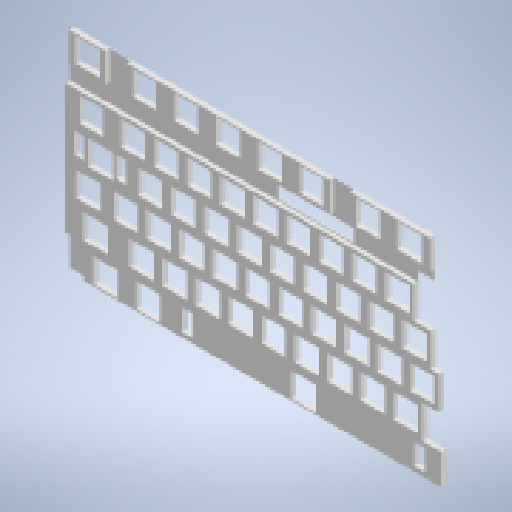
# Autodesk Inventor part: Left plate
Saved by Autodesk Inventor 2025 (Build 290162000, 162)
## iProperties
Created: 2024-08-01
Part Number: Left plate
Material: PET Plastic
Document SubType Name: Modeling
Designer: adam
Density: 1.541 g/cm^3
Appearance: White
Author: adam
Autodesk Inventor part; units mm, degrees
(part 1 of 2)
ref_plane "YZ Plane" through (0, 0, 0) normal (1, 0, 0) x (0, 1, 0)
ref_plane "XZ Plane" through (0, 0, 0) normal (0, 1, 0) x (-1, 0, 0)
ref_plane "XY Plane" through (0, 0, 0) normal (0, 0, 1) x (1, 0, 0)
sketch "Sketch3" plane through (0, 0, 0) normal (0, 0, 1) x (1, 0, 0)
  line L0 (316, -123) -> (0, -123) construction
  line L1 (316, -2) -> (316, -123) construction
  line L2 (0, -2) -> (316, -2) construction
  line L3 (0, -123) -> (0, -2) construction
  circle A0 centre (18.6, -119.6) radius 0.725 construction
  circle A1 centre (23, -114.9) radius 2.55 construction
  circle A2 centre (25.6, -120.65) radius 0.725 construction
  circle A3 centre (43.1, -119.6) radius 0.725 construction
  circle A4 centre (50.1, -120.65) radius 0.725 construction
  circle A5 centre (47.5, -114.9) radius 2.55 construction
  line L4 (67.3517, -120.975) -> (73.3517, -120.975) construction
  line L5 (67.3517, -105.975) -> (67.3517, -120.975) construction
  line L6 (73.3517, -105.975) -> (67.3517, -105.975) construction
  line L7 (73.3517, -120.975) -> (73.3517, -105.975) construction
  circle A6 centre (13.1, -100.5) radius 0.725 construction
  circle A7 centre (20.1, -101.55) radius 0.725 construction
  circle A8 centre (39.35, -100.5) radius 0.725 construction
  circle A9 centre (17.5, -95.8) radius 2.55 construction
  circle A10 centre (46.35, -101.55) radius 0.725 construction
  circle A11 centre (58.35, -100.5) radius 0.725 construction
  circle A12 centre (65.35, -101.55) radius 0.725 construction
  circle A13 centre (77.35, -100.5) radius 0.725 construction
  circle A14 centre (43.75, -95.8) radius 2.55 construction
  circle A15 centre (62.75, -95.8) radius 2.55 construction
  circle A16 centre (81.75, -95.8) radius 2.55 construction
  circle A17 centre (132.4518, -119.675) radius 0.725 construction
  circle A18 centre (139.4518, -120.725) radius 0.725 construction
  circle A19 centre (136.8518, -114.975) radius 2.55 construction
  circle A20 centre (84.35, -101.55) radius 0.725 construction
  circle A21 centre (96.35, -100.5) radius 0.725 construction
  circle A22 centre (103.35, -101.55) radius 0.725 construction
  circle A23 centre (115.35, -100.5) radius 0.725 construction
  circle A24 centre (100.75, -95.8) radius 2.55 construction
  circle A25 centre (119.75, -95.8) radius 2.55 construction
  circle A26 centre (122.35, -101.55) radius 0.725 construction
  circle A27 centre (134.35, -100.5) radius 0.725 construction
  circle A28 centre (141.35, -101.55) radius 0.725 construction
  circle A29 centre (153.35, -100.5) radius 0.725 construction
  circle A30 centre (138.75, -95.8) radius 2.55 construction
  circle A31 centre (157.75, -95.8) radius 2.55 construction
  circle A32 centre (15.6, -82.45) radius 0.725 construction
  circle A33 centre (8.6, -81.4) radius 0.725 construction
  circle A34 centre (37.1, -82.45) radius 0.725 construction
  circle A35 centre (30.1, -81.4) radius 0.725 construction
  circle A36 centre (56.1, -82.45) radius 0.725 construction
  circle A37 centre (49.1, -81.4) radius 0.725 construction
  circle A38 centre (75.1, -82.45) radius 0.725 construction
  circle A39 centre (68.1, -81.4) radius 0.725 construction
  circle A40 centre (13, -76.7) radius 2.55 construction
  circle A41 centre (34.5, -76.7) radius 2.55 construction
  circle A42 centre (53.5, -76.7) radius 2.55 construction
  circle A43 centre (72.5, -76.7) radius 2.55 construction
  circle A44 centre (94.1, -82.45) radius 0.725 construction
  circle A45 centre (87.1, -81.4) radius 0.725 construction
  circle A46 centre (113.1, -82.45) radius 0.725 construction
  circle A47 centre (106.1, -81.4) radius 0.725 construction
  circle A48 centre (132.1, -82.45) radius 0.725 construction
  circle A49 centre (125.1, -81.4) radius 0.725 construction
  circle A50 centre (151.1, -82.45) radius 0.725 construction
  circle A51 centre (144.1, -81.4) radius 0.725 construction
  circle A52 centre (91.5, -76.7) radius 2.55 construction
  circle A53 centre (110.5, -76.7) radius 2.55 construction
  circle A54 centre (129.5, -76.7) radius 2.55 construction
  circle A55 centre (148.5, -76.7) radius 2.55 construction
  circle A56 centre (221.85, -119.6) radius 0.725 construction
  circle A57 centre (228.85, -120.65) radius 0.725 construction
  circle A58 centre (226.25, -114.9) radius 2.55 construction
  line L8 (200.3518, -120.975) -> (206.3518, -120.975) construction
  line L9 (200.3518, -105.975) -> (200.3518, -120.975) construction
  line L10 (206.3518, -105.975) -> (200.3518, -105.975) construction
  line L11 (206.3518, -120.975) -> (206.3518, -105.975) construction
  circle A59 centre (160.35, -101.55) radius 0.725 construction
  circle A60 centre (172.35, -100.5) radius 0.725 construction
  circle A61 centre (179.35, -101.55) radius 0.725 construction
  circle A62 centre (191.35, -100.5) radius 0.725 construction
  circle A63 centre (198.35, -101.55) radius 0.725 construction
  circle A64 centre (176.75, -95.8) radius 2.55 construction
  circle A65 centre (195.75, -95.8) radius 2.55 construction
  circle A66 centre (210.35, -100.5) radius 0.725 construction
  circle A67 centre (217.35, -101.55) radius 0.725 construction
  circle A68 centre (229.35, -100.5) radius 0.725 construction
  circle A69 centre (236.35, -101.55) radius 0.725 construction
  circle A70 centre (214.75, -95.8) radius 2.55 construction
  circle A71 centre (233.75, -95.8) radius 2.55 construction
  circle A72 centre (243.85, -119.6) radius 0.725 construction
  circle A73 centre (250.85, -120.65) radius 0.725 construction
  circle A74 centre (248.25, -114.9) radius 2.55 construction
  circle A75 centre (262.85, -119.6) radius 0.725 construction
  circle A76 centre (269.85, -120.65) radius 0.725 construction
  circle A77 centre (267.25, -114.9) radius 2.55 construction
  circle A78 centre (281.85, -119.6) radius 0.725 construction
  circle A79 centre (288.85, -120.65) radius 0.725 construction
  circle A80 centre (286.25, -114.9) radius 2.55 construction
  circle A81 centre (300.85, -119.6) radius 0.725 construction
  circle A82 centre (307.85, -120.65) radius 0.725 construction
  circle A83 centre (305.25, -114.9) radius 2.55 construction
  circle A84 centre (255.6, -100.5) radius 0.725 construction
  circle A85 centre (262.6, -101.55) radius 0.725 construction
  circle A86 centre (260, -95.8) radius 2.55 construction
  circle A87 centre (281.85, -100.5) radius 0.725 construction
  circle A88 centre (288.85, -101.55) radius 0.725 construction
  circle A89 centre (314, -102.5) radius 0.5 construction
  circle A90 centre (286.25, -95.8) radius 2.55 construction
  circle A91 centre (314, -99.96) radius 0.5 construction
  circle A92 centre (314, -97.42) radius 0.5 construction
  circle A93 centre (314, -94.88) radius 0.5 construction
  circle A94 centre (170.1, -82.45) radius 0.725 construction
  circle A95 centre (163.1, -81.4) radius 0.725 construction
  circle A96 centre (189.1, -82.45) radius 0.725 construction
  circle A97 centre (182.1, -81.4) radius 0.725 construction
  circle A98 centre (208.1, -82.45) radius 0.725 construction
  circle A99 centre (201.1, -81.4) radius 0.725 construction
  circle A100 centre (227.1, -82.45) radius 0.725 construction
  circle A101 centre (220.1, -81.4) radius 0.725 construction
  circle A102 centre (167.5, -76.7) radius 2.55 construction
  circle A103 centre (186.5, -76.7) radius 2.55 construction
  circle A104 centre (205.5, -76.7) radius 2.55 construction
  circle A105 centre (224.5, -76.7) radius 2.55 construction
  circle A106 centre (246.1, -82.45) radius 0.725 construction
  circle A107 centre (239.1, -81.4) radius 0.725 construction
  circle A108 centre (265.1, -82.45) radius 0.725 construction
  circle A109 centre (258.1, -81.4) radius 0.725 construction
  circle A110 centre (314, -92.34) radius 0.5 construction
  circle A111 centre (314, -89.8) radius 0.5 construction
  line L12 (275, -82.25) -> (290, -82.25) construction
  line L13 (275, -76.25) -> (275, -82.25) construction
  line L14 (290, -76.25) -> (275, -76.25) construction
  line L15 (290, -82.25) -> (290, -76.25) construction
  circle A112 centre (243.5, -76.7) radius 2.55 construction
  circle A113 centre (262.5, -76.7) radius 2.55 construction
  circle A114 centre (288.675, -71.675) radius 0.725 construction
  circle A115 centre (283.975, -67.275) radius 2.55 construction
  circle A116 centre (289.725, -64.675) radius 0.725 construction
  circle A117 centre (22.6, -63.35) radius 0.725 construction
  circle A118 centre (15.6, -62.3) radius 0.725 construction
  circle A119 centre (20, -57.6) radius 2.55 construction
  line L16 (5, -63.6) -> (11, -63.6) construction
  line L17 (5, -48.6) -> (5, -63.6) construction
  line L18 (11, -48.6) -> (5, -48.6) construction
  line L19 (11, -63.6) -> (11, -48.6) construction
  line L20 (29, -63.6) -> (35, -63.6) construction
  line L21 (29, -48.6) -> (29, -63.6) construction
  line L22 (35, -48.6) -> (29, -48.6) construction
  line L23 (35, -63.6) -> (35, -48.6) construction
  circle A120 centre (51.35, -63.35) radius 0.725 construction
  circle A121 centre (44.35, -62.3) radius 0.725 construction
  circle A122 centre (48.75, -57.6) radius 2.55 construction
  circle A123 centre (70.35, -63.35) radius 0.725 construction
  circle A124 centre (63.35, -62.3) radius 0.725 construction
  circle A125 centre (82.35, -62.3) radius 0.725 construction
  circle A126 centre (67.75, -57.6) radius 2.55 construction
  circle A127 centre (10.6, -43.2) radius 0.725 construction
  circle A128 centre (17.6, -44.25) radius 0.725 construction
  circle A129 centre (34.6, -43.2) radius 0.725 construction
  circle A130 centre (41.6, -44.25) radius 0.725 construction
  circle A131 centre (15, -38.5) radius 2.55 construction
  circle A132 centre (39, -38.5) radius 2.55 construction
  circle A133 centre (53.6, -43.2) radius 0.725 construction
  circle A134 centre (60.6, -44.25) radius 0.725 construction
  circle A135 centre (72.6, -43.2) radius 0.725 construction
  circle A136 centre (79.6, -44.25) radius 0.725 construction
  circle A137 centre (58, -38.5) radius 2.55 construction
  circle A138 centre (77, -38.5) radius 2.55 construction
  circle A139 centre (89.35, -63.35) radius 0.725 construction
  circle A140 centre (101.35, -62.3) radius 0.725 construction
  circle A141 centre (86.75, -57.6) radius 2.55 construction
  circle A142 centre (108.35, -63.35) radius 0.725 construction
  circle A143 centre (120.35, -62.3) radius 0.725 construction
  circle A144 centre (105.75, -57.6) radius 2.55 construction
  circle A145 centre (127.35, -63.35) radius 0.725 construction
  circle A146 centre (139.35, -62.3) radius 0.725 construction
  circle A147 centre (124.75, -57.6) radius 2.55 construction
  circle A148 centre (146.35, -63.35) radius 0.725 construction
  circle A149 centre (158.35, -62.3) radius 0.725 construction
  circle A150 centre (143.75, -57.6) radius 2.55 construction
  circle A151 centre (91.6, -43.2) radius 0.725 construction
  circle A152 centre (98.6, -44.25) radius 0.725 construction
  circle A153 centre (110.6, -43.2) radius 0.725 construction
  circle A154 centre (117.6, -44.25) radius 0.725 construction
  circle A155 centre (96, -38.5) radius 2.55 construction
  circle A156 centre (115, -38.5) radius 2.55 construction
  circle A157 centre (129.6, -43.2) radius 0.725 construction
  circle A158 centre (136.6, -44.25) radius 0.725 construction
  circle A159 centre (148.6, -43.2) radius 0.725 construction
  circle A160 centre (155.6, -44.25) radius 0.725 construction
  circle A161 centre (134, -38.5) radius 2.55 construction
  circle A162 centre (153, -38.5) radius 2.55 construction
  circle A163 centre (8.1, -14.7) radius 0.725 construction
  circle A164 centre (15.1, -15.75) radius 0.725 construction
  circle A165 centre (41.1, -14.7) radius 0.725 construction
  circle A166 centre (12.5, -10) radius 2.55 construction
  circle A167 centre (48.1, -15.75) radius 0.725 construction
  circle A168 centre (65.1, -14.7) radius 0.725 construction
  circle A169 centre (72.1, -15.75) radius 0.725 construction
  circle A170 centre (45.5, -10) radius 2.55 construction
  circle A171 centre (69.5, -10) radius 2.55 construction
  circle A172 centre (123.5, -26.25) radius 0.425 construction
  circle A173 centre (126, -26.25) radius 0.425 construction
  circle A174 centre (128.5, -26.25) radius 0.425 construction
  circle A175 centre (131, -26.25) radius 0.425 construction
  circle A176 centre (133.5, -26.25) radius 0.425 construction
  circle A177 centre (136, -26.25) radius 0.425 construction
  circle A178 centre (138.5, -26.25) radius 0.425 construction
  circle A179 centre (122.25, -23.75) radius 0.425 construction
  circle A180 centre (124.75, -23.75) radius 0.425 construction
  circle A181 centre (127.25, -23.75) radius 0.425 construction
  circle A182 centre (129.75, -23.75) radius 0.425 construction
  circle A183 centre (132.25, -23.75) radius 0.425 construction
  circle A184 centre (134.75, -23.75) radius 0.425 construction
  circle A185 centre (137.25, -23.75) radius 0.425 construction
  circle A186 centre (139.75, -23.75) radius 0.425 construction
  circle A187 centre (141, -26.25) radius 0.425 construction
  circle A188 centre (143.5, -26.25) radius 0.425 construction
  circle A189 centre (146, -26.25) radius 0.425 construction
  circle A190 centre (148.5, -26.25) radius 0.425 construction
  circle A191 centre (151, -26.25) radius 0.425 construction
  circle A192 centre (153.5, -26.25) radius 0.425 construction
  circle A193 centre (156, -26.25) radius 0.425 construction
  circle A194 centre (158.5, -26.25) radius 0.425 construction
  circle A195 centre (142.25, -23.75) radius 0.425 construction
  circle A196 centre (144.75, -23.75) radius 0.425 construction
  circle A197 centre (147.25, -23.75) radius 0.425 construction
  circle A198 centre (149.75, -23.75) radius 0.425 construction
  circle A199 centre (152.25, -23.75) radius 0.425 construction
  circle A200 centre (154.75, -23.75) radius 0.425 construction
  circle A201 centre (157.25, -23.75) radius 0.425 construction
  circle A202 centre (89.1, -14.7) radius 0.725 construction
  circle A203 centre (96.1, -15.75) radius 0.725 construction
  circle A204 centre (113.1, -14.7) radius 0.725 construction
  circle A205 centre (120.1, -15.75) radius 0.725 construction
  circle A206 centre (93.5, -10) radius 2.55 construction
  circle A207 centre (117.5, -10) radius 2.55 construction
  circle A208 centre (137.1, -14.7) radius 0.725 construction
  circle A209 centre (144.1, -15.75) radius 0.725 construction
  circle A210 centre (141.5, -10) radius 2.55 construction
  circle A211 centre (165.35, -63.35) radius 0.725 construction
  circle A212 centre (177.35, -62.3) radius 0.725 construction
  circle A213 centre (162.75, -57.6) radius 2.55 construction
  circle A214 centre (184.35, -63.35) radius 0.725 construction
  circle A215 centre (196.35, -62.3) radius 0.725 construction
  circle A216 centre (181.75, -57.6) radius 2.55 construction
  circle A217 centre (203.35, -63.35) radius 0.725 construction
  circle A218 centre (215.35, -62.3) radius 0.725 construction
  circle A219 centre (200.75, -57.6) radius 2.55 construction
  circle A220 centre (222.35, -63.35) radius 0.725 construction
  circle A221 centre (234.35, -62.45) radius 0.725 construction
  circle A222 centre (219.75, -57.6) radius 2.55 construction
  circle A223 centre (167.6, -43.2) radius 0.725 construction
  circle A224 centre (174.6, -44.25) radius 0.725 construction
  circle A225 centre (186.6, -43.2) radius 0.725 construction
  circle A226 centre (193.6, -44.25) radius 0.725 construction
  circle A227 centre (172, -38.5) radius 2.55 construction
  circle A228 centre (191, -38.5) radius 2.55 construction
  circle A229 centre (205.6, -43.2) radius 0.725 construction
  circle A230 centre (212.6, -44.25) radius 0.725 construction
  circle A231 centre (224.6, -43.2) radius 0.725 construction
  circle A232 centre (231.6, -44.25) radius 0.725 construction
  circle A233 centre (210, -38.5) radius 2.55 construction
  circle A234 centre (229, -38.5) radius 2.55 construction
  circle A235 centre (241.35, -63.5) radius 0.725 construction
  circle A236 centre (253.35, -62.4466) radius 0.725 construction
  circle A237 centre (238.75, -57.75) radius 2.55 construction
  circle A238 centre (260.35, -63.4966) radius 0.725 construction
  circle A239 centre (257.75, -57.7466) radius 2.55 construction
  line L24 (275, -58.25) -> (290, -58.25) construction
  line L25 (275, -52.25) -> (275, -58.25) construction
  line L26 (290, -52.25) -> (275, -52.25) construction
  line L27 (290, -58.25) -> (290, -52.25) construction
  circle A240 centre (243.6, -43.2) radius 0.725 construction
  circle A241 centre (250.6, -44.25) radius 0.725 construction
  circle A242 centre (262.6, -43.2) radius 0.725 construction
  circle A243 centre (269.6, -44.25) radius 0.725 construction
  circle A244 centre (248, -38.5) radius 2.55 construction
  circle A245 centre (267, -38.5) radius 2.55 construction
  circle A246 centre (281.6, -43.2) radius 0.725 construction
  circle A247 centre (288.6, -44.25) radius 0.725 construction
  circle A248 centre (300.6, -43.2) radius 0.725 construction
  circle A249 centre (307.6, -44.25) radius 0.725 construction
  circle A250 centre (286, -38.5) radius 2.55 construction
  circle A251 centre (305, -38.5) radius 2.55 construction
  circle A252 centre (161, -26.25) radius 0.425 construction
  circle A253 centre (159.75, -23.75) radius 0.425 construction
  circle A254 centre (219, -34) radius 1.6 construction
  circle A255 centre (169.6, -14.7) radius 0.725 construction
  circle A256 centre (176.6, -15.75) radius 0.725 construction
  circle A257 centre (193.6, -14.7) radius 0.725 construction
  circle A258 centre (174, -10) radius 2.55 construction
  circle A259 centre (198, -10) radius 2.55 construction
  circle A260 centre (200.6, -15.75) radius 0.725 construction
  circle A261 centre (217.6, -14.7) radius 0.725 construction
  circle A262 centre (224.6, -15.75) radius 0.725 construction
  circle A263 centre (222, -10) radius 2.55 construction
  circle A264 centre (241.6, -14.7) radius 0.725 construction
  circle A265 centre (248.6, -15.75) radius 0.725 construction
  circle A266 centre (265.6, -14.7) radius 0.725 construction
  circle A267 centre (272.6, -15.75) radius 0.725 construction
  circle A268 centre (246, -10) radius 2.55 construction
  circle A269 centre (270, -10) radius 2.55 construction
  circle A270 centre (299.1, -14.7) radius 0.725 construction
  circle A271 centre (306.1, -15.75) radius 0.725 construction
  circle A272 centre (303.5, -10) radius 2.55 construction
  line L28 (216.3009, -122.9025) -> (216.3009, -103.8025)
  line L29 (216.3009, -103.8025) -> (205.25, -103.8025)
  line L30 (205.25, -103.8025) -> (205.25, -86.25)
  line L31 (205.25, -86.25) -> (215, -86.25)
  line L32 (215, -86.25) -> (215, -67.15)
  line L33 (215, -67.15) -> (210.25, -67.15)
  line L34 (210.25, -67.15) -> (210.25, -48.05)
  line L35 (210.25, -48.05) -> (200.5, -48.05)
  line L36 (200.5, -48.05) -> (200.5, -24.25)
  line L37 (200.5, -24.25) -> (210, -24.25)
  line L38 (210, -24.25) -> (210, -1.9975)
  line L39 (198, -10) -> (210, -10) construction
  line L40 (210, -10) -> (222, -10) construction
  line L41 (191, -38.5) -> (200.5, -38.5) construction
  line L42 (210, -38.5) -> (200.5, -38.5) construction
  line L43 (200.75, -57.6) -> (210.25, -57.6) construction
  line L44 (219.75, -57.6) -> (210.25, -57.6) construction
  line L45 (205.5, -76.7) -> (215, -76.7) construction
  line L46 (224.5, -76.7) -> (215, -76.7) construction
  line L47 (195.75, -95.8) -> (205.25, -95.8) construction
  line L48 (214.75, -95.8) -> (205.25, -95.8) construction
  line L49 (226.25, -114.9) -> (216.3009, -114.9) construction
  line L50 (206.3518, -114.9) -> (216.3009, -114.9) construction
  line L51 (204, -10) -> (204, -24.25) construction
  line L52 (204, -38.5) -> (204, -24.25) construction
  line L53 (206.8595, -38.5) -> (206.8595, -48.05) construction
  line L54 (206.8595, -57.6) -> (206.8595, -48.05) construction
  line L55 (211.5322, -57.6) -> (211.5322, -67.15) construction
  line L56 (211.5322, -67.15) -> (211.5322, -76.7) construction
  line L57 (209.7471, -76.7) -> (209.7471, -86.25) construction
  line L58 (209.7471, -86.25) -> (209.7471, -95.8) construction
  line L59 (207.7475, -88.7975) -> (221.7525, -88.7975) construction
  line L60 (221.7525, -88.7975) -> (221.7525, -102.8025) construction
  line L61 (221.7525, -102.8025) -> (207.7475, -102.8025) construction
  line L62 (207.7475, -102.8025) -> (207.7475, -88.7975) construction
  line L63 (207.7475, -88.7975) -> (221.7525, -102.8025) construction
  line L64 (221.7525, -88.7975) -> (207.7475, -102.8025) construction
  line L65 (129.8493, -107.9725) -> (143.8543, -107.9725)
  line L66 (143.8543, -107.9725) -> (143.8543, -121.9775)
  line L67 (143.8543, -121.9775) -> (129.8493, -121.9775)
  line L68 (129.8493, -121.9775) -> (129.8493, -107.9725)
  line L69 (129.8493, -107.9725) -> (143.8543, -121.9775) construction
  line L70 (143.8543, -107.9725) -> (129.8493, -121.9775) construction
  line L71 (143.8543, -107.9725) -> (216.3009, -107.9725) construction
  line L72 (5.4975, -2.9975) -> (19.5025, -2.9975)
  line L73 (19.5025, -2.9975) -> (19.5025, -17.0025)
  line L74 (19.5025, -17.0025) -> (5.4975, -17.0025)
  line L75 (5.4975, -17.0025) -> (5.4975, -2.9975)
  line L76 (5.4975, -2.9975) -> (19.5025, -17.0025) construction
  line L77 (19.5025, -2.9975) -> (5.4975, -17.0025) construction
  line L78 (38.4975, -2.9975) -> (52.5025, -2.9975)
  line L79 (52.5025, -2.9975) -> (52.5025, -17.0025)
  line L80 (52.5025, -17.0025) -> (38.4975, -17.0025)
  line L81 (38.4975, -17.0025) -> (38.4975, -2.9975)
  line L82 (38.4975, -2.9975) -> (52.5025, -17.0025) construction
  line L83 (52.5025, -2.9975) -> (38.4975, -17.0025) construction
  line L84 (62.4975, -2.9975) -> (76.5025, -2.9975)
  line L85 (76.5025, -2.9975) -> (76.5025, -17.0025)
  line L86 (76.5025, -17.0025) -> (62.4975, -17.0025)
  line L87 (62.4975, -17.0025) -> (62.4975, -2.9975)
  line L88 (62.4975, -2.9975) -> (76.5025, -17.0025) construction
  line L89 (76.5025, -2.9975) -> (62.4975, -17.0025) construction
  line L90 (86.4975, -2.9975) -> (100.5025, -2.9975)
  line L91 (100.5025, -2.9975) -> (100.5025, -17.0025)
  line L92 (100.5025, -17.0025) -> (86.4975, -17.0025)
  line L93 (86.4975, -17.0025) -> (86.4975, -2.9975)
  line L94 (86.4975, -2.9975) -> (100.5025, -17.0025) construction
  line L95 (100.5025, -2.9975) -> (86.4975, -17.0025) construction
  line L96 (110.4975, -2.9975) -> (124.5025, -2.9975)
  line L97 (124.5025, -2.9975) -> (124.5025, -17.0025)
  line L98 (124.5025, -17.0025) -> (110.4975, -17.0025)
  line L99 (110.4975, -17.0025) -> (110.4975, -2.9975)
  line L100 (110.4975, -2.9975) -> (124.5025, -17.0025) construction
  line L101 (124.5025, -2.9975) -> (110.4975, -17.0025) construction
  line L102 (134.4975, -2.9975) -> (148.5025, -2.9975)
  line L103 (148.5025, -2.9975) -> (148.5025, -17.0025)
  line L104 (148.5025, -17.0025) -> (134.4975, -17.0025)
  line L105 (134.4975, -17.0025) -> (134.4975, -2.9975)
  line L106 (134.4975, -2.9975) -> (148.5025, -17.0025) construction
  line L107 (148.5025, -2.9975) -> (134.4975, -17.0025) construction
  line L108 (166.9975, -2.9975) -> (181.0025, -2.9975)
  line L109 (181.0025, -2.9975) -> (181.0025, -17.0025)
  line L110 (181.0025, -17.0025) -> (166.9975, -17.0025)
  line L111 (166.9975, -17.0025) -> (166.9975, -2.9975)
  line L112 (166.9975, -2.9975) -> (181.0025, -17.0025) construction
  line L113 (181.0025, -2.9975) -> (166.9975, -17.0025) construction
  line L114 (190.9975, -2.9975) -> (205.0025, -2.9975)
  line L115 (205.0025, -2.9975) -> (205.0025, -17.0025)
  line L116 (205.0025, -17.0025) -> (190.9975, -17.0025)
  line L117 (190.9975, -17.0025) -> (190.9975, -2.9975)
  line L118 (190.9975, -2.9975) -> (205.0025, -17.0025) construction
  line L119 (205.0025, -2.9975) -> (190.9975, -17.0025) construction
  line L120 (7.9975, -31.4975) -> (22.0025, -31.4975)
  line L121 (22.0025, -31.4975) -> (22.0025, -45.5025)
  line L122 (22.0025, -45.5025) -> (7.9975, -45.5025)
  line L123 (7.9975, -45.5025) -> (7.9975, -31.4975)
  line L124 (7.9975, -31.4975) -> (22.0025, -45.5025) construction
  line L125 (22.0025, -31.4975) -> (7.9975, -45.5025) construction
  line L126 (31.9975, -31.4975) -> (46.0025, -31.4975)
  line L127 (46.0025, -31.4975) -> (46.0025, -45.5025)
  line L128 (46.0025, -45.5025) -> (31.9975, -45.5025)
  line L129 (31.9975, -45.5025) -> (31.9975, -31.4975)
  line L130 (31.9975, -31.4975) -> (46.0025, -45.5025) construction
  line L131 (46.0025, -31.4975) -> (31.9975, -45.5025) construction
  line L132 (50.9975, -31.4975) -> (65.0025, -31.4975)
  line L133 (65.0025, -31.4975) -> (65.0025, -45.5025)
  line L134 (65.0025, -45.5025) -> (50.9975, -45.5025)
  line L135 (50.9975, -45.5025) -> (50.9975, -31.4975)
  line L136 (50.9975, -31.4975) -> (65.0025, -45.5025) construction
  line L137 (65.0025, -31.4975) -> (50.9975, -45.5025) construction
  line L138 (69.9975, -31.4975) -> (84.0025, -31.4975)
  line L139 (84.0025, -31.4975) -> (84.0025, -45.5025)
  line L140 (84.0025, -45.5025) -> (69.9975, -45.5025)
  line L141 (69.9975, -45.5025) -> (69.9975, -31.4975)
  line L142 (69.9975, -31.4975) -> (84.0025, -45.5025) construction
  line L143 (84.0025, -31.4975) -> (69.9975, -45.5025) construction
  line L144 (88.9975, -31.4975) -> (103.0025, -31.4975)
  line L145 (103.0025, -31.4975) -> (103.0025, -45.5025)
  line L146 (103.0025, -45.5025) -> (88.9975, -45.5025)
  line L147 (88.9975, -45.5025) -> (88.9975, -31.4975)
  line L148 (88.9975, -31.4975) -> (103.0025, -45.5025) construction
  line L149 (103.0025, -31.4975) -> (88.9975, -45.5025) construction
  line L150 (107.9975, -31.4975) -> (122.0025, -31.4975)
  line L151 (122.0025, -31.4975) -> (122.0025, -45.5025)
  line L152 (122.0025, -45.5025) -> (107.9975, -45.5025)
  line L153 (107.9975, -45.5025) -> (107.9975, -31.4975)
  line L154 (107.9975, -31.4975) -> (122.0025, -45.5025) construction
  line L155 (122.0025, -31.4975) -> (107.9975, -45.5025) construction
  line L156 (126.9975, -31.4975) -> (141.0025, -31.4975)
  line L157 (141.0025, -31.4975) -> (141.0025, -45.5025)
  line L158 (141.0025, -45.5025) -> (126.9975, -45.5025)
  line L159 (126.9975, -45.5025) -> (126.9975, -31.4975)
  line L160 (126.9975, -31.4975) -> (141.0025, -45.5025) construction
  line L161 (141.0025, -31.4975) -> (126.9975, -45.5025) construction
  line L162 (145.9975, -31.4975) -> (160.0025, -31.4975)
  line L163 (160.0025, -31.4975) -> (160.0025, -45.5025)
  line L164 (160.0025, -45.5025) -> (145.9975, -45.5025)
  line L165 (145.9975, -45.5025) -> (145.9975, -31.4975)
  line L166 (145.9975, -31.4975) -> (160.0025, -45.5025) construction
  line L167 (160.0025, -31.4975) -> (145.9975, -45.5025) construction
  line L168 (164.9975, -31.4975) -> (179.0025, -31.4975)
  line L169 (179.0025, -31.4975) -> (179.0025, -45.5025)
  line L170 (179.0025, -45.5025) -> (164.9975, -45.5025)
  line L171 (164.9975, -45.5025) -> (164.9975, -31.4975)
  line L172 (164.9975, -31.4975) -> (179.0025, -45.5025) construction
  line L173 (179.0025, -31.4975) -> (164.9975, -45.5025) construction
  line L174 (183.9975, -31.4975) -> (198.0025, -31.4975)
  line L175 (198.0025, -31.4975) -> (198.0025, -45.5025)
  line L176 (198.0025, -45.5025) -> (183.9975, -45.5025)
  line L177 (183.9975, -45.5025) -> (183.9975, -31.4975)
  line L178 (183.9975, -31.4975) -> (198.0025, -45.5025) construction
  line L179 (198.0025, -31.4975) -> (183.9975, -45.5025) construction
  line L180 (12.9975, -50.5975) -> (27.0025, -50.5975)
  line L181 (27.0025, -50.5975) -> (27.0025, -64.6025)
  line L182 (27.0025, -64.6025) -> (12.9975, -64.6025)
  line L183 (12.9975, -64.6025) -> (12.9975, -50.5975)
  line L184 (12.9975, -50.5975) -> (27.0025, -64.6025) construction
  line L185 (27.0025, -50.5975) -> (12.9975, -64.6025) construction
  line L186 (41.7475, -50.5975) -> (55.7525, -50.5975)
  line L187 (55.7525, -50.5975) -> (55.7525, -64.6025)
  line L188 (55.7525, -64.6025) -> (41.7475, -64.6025)
  line L189 (41.7475, -64.6025) -> (41.7475, -50.5975)
  line L190 (41.7475, -50.5975) -> (55.7525, -64.6025) construction
  line L191 (55.7525, -50.5975) -> (41.7475, -64.6025) construction
  line L192 (60.7475, -50.5975) -> (74.7525, -50.5975)
  line L193 (74.7525, -50.5975) -> (74.7525, -64.6025)
  line L194 (74.7525, -64.6025) -> (60.7475, -64.6025)
  line L195 (60.7475, -64.6025) -> (60.7475, -50.5975)
  line L196 (60.7475, -50.5975) -> (74.7525, -64.6025) construction
  line L197 (74.7525, -50.5975) -> (60.7475, -64.6025) construction
  line L198 (79.7475, -50.5975) -> (93.7525, -50.5975)
  line L199 (93.7525, -50.5975) -> (93.7525, -64.6025)
  line L200 (93.7525, -64.6025) -> (79.7475, -64.6025)
  line L201 (79.7475, -64.6025) -> (79.7475, -50.5975)
  line L202 (79.7475, -50.5975) -> (93.7525, -64.6025) construction
  line L203 (93.7525, -50.5975) -> (79.7475, -64.6025) construction
  line L204 (98.7475, -50.5975) -> (112.7525, -50.5975)
  line L205 (112.7525, -50.5975) -> (112.7525, -64.6025)
  line L206 (112.7525, -64.6025) -> (98.7475, -64.6025)
  line L207 (98.7475, -64.6025) -> (98.7475, -50.5975)
  line L208 (98.7475, -50.5975) -> (112.7525, -64.6025) construction
  line L209 (112.7525, -50.5975) -> (98.7475, -64.6025) construction
  line L210 (117.7475, -50.5975) -> (131.7525, -50.5975)
  line L211 (131.7525, -50.5975) -> (131.7525, -64.6025)
  line L212 (131.7525, -64.6025) -> (117.7475, -64.6025)
  line L213 (117.7475, -64.6025) -> (117.7475, -50.5975)
  line L214 (117.7475, -50.5975) -> (131.7525, -64.6025) construction
  line L215 (131.7525, -50.5975) -> (117.7475, -64.6025) construction
  line L216 (136.7475, -50.5975) -> (150.7525, -50.5975)
  line L217 (150.7525, -50.5975) -> (150.7525, -64.6025)
  line L218 (150.7525, -64.6025) -> (136.7475, -64.6025)
  line L219 (136.7475, -64.6025) -> (136.7475, -50.5975)
  line L220 (136.7475, -50.5975) -> (150.7525, -64.6025) construction
  line L221 (150.7525, -50.5975) -> (136.7475, -64.6025) construction
  line L222 (155.7475, -50.5975) -> (169.7525, -50.5975)
  line L223 (169.7525, -50.5975) -> (169.7525, -64.6025)
  line L224 (169.7525, -64.6025) -> (155.7475, -64.6025)
  line L225 (155.7475, -64.6025) -> (155.7475, -50.5975)
  line L226 (155.7475, -50.5975) -> (169.7525, -64.6025) construction
  line L227 (169.7525, -50.5975) -> (155.7475, -64.6025) construction
  line L228 (174.7475, -50.5975) -> (188.7525, -50.5975)
  line L229 (188.7525, -50.5975) -> (188.7525, -64.6025)
  line L230 (188.7525, -64.6025) -> (174.7475, -64.6025)
  line L231 (174.7475, -64.6025) -> (174.7475, -50.5975)
  line L232 (174.7475, -50.5975) -> (188.7525, -64.6025) construction
  line L233 (188.7525, -50.5975) -> (174.7475, -64.6025) construction
  line L234 (193.7475, -50.5975) -> (207.7525, -50.5975)
  line L235 (207.7525, -50.5975) -> (207.7525, -64.6025)
  line L236 (207.7525, -64.6025) -> (193.7475, -64.6025)
  line L237 (193.7475, -64.6025) -> (193.7475, -50.5975)
  line L238 (193.7475, -50.5975) -> (207.7525, -64.6025) construction
  line L239 (207.7525, -50.5975) -> (193.7475, -64.6025) construction
  line L240 (198.4975, -69.6975) -> (212.5025, -69.6975)
  line L241 (212.5025, -69.6975) -> (212.5025, -83.7025)
  line L242 (212.5025, -83.7025) -> (198.4975, -83.7025)
  line L243 (198.4975, -83.7025) -> (198.4975, -69.6975)
  line L244 (198.4975, -69.6975) -> (212.5025, -83.7025) construction
  line L245 (212.5025, -69.6975) -> (198.4975, -83.7025) construction
  line L246 (179.4975, -69.6975) -> (193.5025, -69.6975)
  line L247 (193.5025, -69.6975) -> (193.5025, -83.7025)
  line L248 (193.5025, -83.7025) -> (179.4975, -83.7025)
  line L249 (179.4975, -83.7025) -> (179.4975, -69.6975)
  line L250 (179.4975, -69.6975) -> (193.5025, -83.7025) construction
  line L251 (193.5025, -69.6975) -> (179.4975, -83.7025) construction
  line L252 (160.4975, -69.6975) -> (174.5025, -69.6975)
  line L253 (174.5025, -69.6975) -> (174.5025, -83.7025)
  line L254 (174.5025, -83.7025) -> (160.4975, -83.7025)
  line L255 (160.4975, -83.7025) -> (160.4975, -69.6975)
  line L256 (160.4975, -69.6975) -> (174.5025, -83.7025) construction
  line L257 (174.5025, -69.6975) -> (160.4975, -83.7025) construction
  line L258 (141.4975, -69.6975) -> (155.5025, -69.6975)
  line L259 (155.5025, -69.6975) -> (155.5025, -83.7025)
  line L260 (155.5025, -83.7025) -> (141.4975, -83.7025)
  line L261 (141.4975, -83.7025) -> (141.4975, -69.6975)
  line L262 (141.4975, -69.6975) -> (155.5025, -83.7025) construction
  line L263 (155.5025, -69.6975) -> (141.4975, -83.7025) construction
  line L264 (122.4975, -69.6975) -> (136.5025, -69.6975)
  line L265 (136.5025, -69.6975) -> (136.5025, -83.7025)
  line L266 (136.5025, -83.7025) -> (122.4975, -83.7025)
  line L267 (122.4975, -83.7025) -> (122.4975, -69.6975)
  line L268 (122.4975, -69.6975) -> (136.5025, -83.7025) construction
  line L269 (136.5025, -69.6975) -> (122.4975, -83.7025) construction
  line L270 (103.4975, -69.6975) -> (117.5025, -69.6975)
  line L271 (117.5025, -69.6975) -> (117.5025, -83.7025)
  line L272 (117.5025, -83.7025) -> (103.4975, -83.7025)
  line L273 (103.4975, -83.7025) -> (103.4975, -69.6975)
  line L274 (103.4975, -69.6975) -> (117.5025, -83.7025) construction
  line L275 (117.5025, -69.6975) -> (103.4975, -83.7025) construction
  line L276 (84.4975, -69.6975) -> (98.5025, -69.6975)
  line L277 (98.5025, -69.6975) -> (98.5025, -83.7025)
  line L278 (98.5025, -83.7025) -> (84.4975, -83.7025)
  line L279 (84.4975, -83.7025) -> (84.4975, -69.6975)
  line L280 (84.4975, -69.6975) -> (98.5025, -83.7025) construction
  line L281 (98.5025, -69.6975) -> (84.4975, -83.7025) construction
  line L282 (65.4975, -69.6975) -> (79.5025, -69.6975)
  line L283 (79.5025, -69.6975) -> (79.5025, -83.7025)
  line L284 (79.5025, -83.7025) -> (65.4975, -83.7025)
  line L285 (65.4975, -83.7025) -> (65.4975, -69.6975)
  line L286 (65.4975, -69.6975) -> (79.5025, -83.7025) construction
  line L287 (79.5025, -69.6975) -> (65.4975, -83.7025) construction
  line L288 (46.4975, -69.6975) -> (60.5025, -69.6975)
  line L289 (60.5025, -69.6975) -> (60.5025, -83.7025)
  line L290 (60.5025, -83.7025) -> (46.4975, -83.7025)
  line L291 (46.4975, -83.7025) -> (46.4975, -69.6975)
  line L292 (46.4975, -69.6975) -> (60.5025, -83.7025) construction
  line L293 (60.5025, -69.6975) -> (46.4975, -83.7025) construction
  line L294 (27.4975, -69.6975) -> (41.5025, -69.6975)
  line L295 (41.5025, -69.6975) -> (41.5025, -83.7025)
  line L296 (41.5025, -83.7025) -> (27.4975, -83.7025)
  line L297 (27.4975, -83.7025) -> (27.4975, -69.6975)
  line L298 (27.4975, -69.6975) -> (41.5025, -83.7025) construction
  line L299 (41.5025, -69.6975) -> (27.4975, -83.7025) construction
  line L300 (5.9975, -69.6975) -> (20.0025, -69.6975)
  line L301 (20.0025, -69.6975) -> (20.0025, -83.7025)
  line L302 (20.0025, -83.7025) -> (5.9975, -83.7025)
  line L303 (5.9975, -83.7025) -> (5.9975, -69.6975)
  line L304 (5.9975, -69.6975) -> (20.0025, -83.7025) construction
  line L305 (20.0025, -69.6975) -> (5.9975, -83.7025) construction
  line L306 (10.4975, -88.7975) -> (24.5025, -88.7975)
  line L307 (24.5025, -88.7975) -> (24.5025, -102.8025)
  line L308 (24.5025, -102.8025) -> (10.4975, -102.8025)
  line L309 (10.4975, -102.8025) -> (10.4975, -88.7975)
  line L310 (10.4975, -88.7975) -> (24.5025, -102.8025) construction
  line L311 (24.5025, -88.7975) -> (10.4975, -102.8025) construction
  line L312 (36.7475, -88.7975) -> (50.7525, -88.7975)
  line L313 (50.7525, -88.7975) -> (50.7525, -102.8025)
  line L314 (50.7525, -102.8025) -> (36.7475, -102.8025)
  line L315 (36.7475, -102.8025) -> (36.7475, -88.7975)
  line L316 (36.7475, -88.7975) -> (50.7525, -102.8025) construction
  line L317 (50.7525, -88.7975) -> (36.7475, -102.8025) construction
  line L318 (55.7475, -88.7975) -> (69.7525, -88.7975)
  line L319 (69.7525, -88.7975) -> (69.7525, -102.8025)
  line L320 (69.7525, -102.8025) -> (55.7475, -102.8025)
  line L321 (55.7475, -102.8025) -> (55.7475, -88.7975)
  line L322 (55.7475, -88.7975) -> (69.7525, -102.8025) construction
  line L323 (69.7525, -88.7975) -> (55.7475, -102.8025) construction
  line L324 (74.7475, -88.7975) -> (88.7525, -88.7975)
  line L325 (88.7525, -88.7975) -> (88.7525, -102.8025)
  line L326 (88.7525, -102.8025) -> (74.7475, -102.8025)
  line L327 (74.7475, -102.8025) -> (74.7475, -88.7975)
  line L328 (74.7475, -88.7975) -> (88.7525, -102.8025) construction
  line L329 (88.7525, -88.7975) -> (74.7475, -102.8025) construction
  line L330 (93.7475, -88.7975) -> (107.7525, -88.7975)
  line L331 (107.7525, -88.7975) -> (107.7525, -102.8025)
  line L332 (107.7525, -102.8025) -> (93.7475, -102.8025)
  line L333 (93.7475, -102.8025) -> (93.7475, -88.7975)
  line L334 (93.7475, -88.7975) -> (107.7525, -102.8025) construction
  line L335 (107.7525, -88.7975) -> (93.7475, -102.8025) construction
  line L336 (112.7475, -88.7975) -> (126.7525, -88.7975)
  line L337 (126.7525, -88.7975) -> (126.7525, -102.8025)
  line L338 (126.7525, -102.8025) -> (112.7475, -102.8025)
  line L339 (112.7475, -102.8025) -> (112.7475, -88.7975)
  line L340 (112.7475, -88.7975) -> (126.7525, -102.8025) construction
  line L341 (126.7525, -88.7975) -> (112.7475, -102.8025) construction
  line L342 (131.7475, -88.7975) -> (145.7525, -88.7975)
  line L343 (145.7525, -88.7975) -> (145.7525, -102.8025)
  line L344 (145.7525, -102.8025) -> (131.7475, -102.8025)
  line L345 (131.7475, -102.8025) -> (131.7475, -88.7975)
  line L346 (131.7475, -88.7975) -> (145.7525, -102.8025) construction
  line L347 (145.7525, -88.7975) -> (131.7475, -102.8025) construction
  line L348 (150.7475, -88.7975) -> (164.7525, -88.7975)
  line L349 (164.7525, -88.7975) -> (164.7525, -102.8025)
  line L350 (164.7525, -102.8025) -> (150.7475, -102.8025)
  line L351 (150.7475, -102.8025) -> (150.7475, -88.7975)
  line L352 (150.7475, -88.7975) -> (164.7525, -102.8025) construction
  line L353 (164.7525, -88.7975) -> (150.7475, -102.8025) construction
  line L354 (169.7475, -88.7975) -> (183.7525, -88.7975)
  line L355 (183.7525, -88.7975) -> (183.7525, -102.8025)
  line L356 (183.7525, -102.8025) -> (169.7475, -102.8025)
  line L357 (169.7475, -102.8025) -> (169.7475, -88.7975)
  line L358 (169.7475, -88.7975) -> (183.7525, -102.8025) construction
  line L359 (183.7525, -88.7975) -> (169.7475, -102.8025) construction
  line L360 (188.7475, -88.7975) -> (202.7525, -88.7975)
  line L361 (202.7525, -88.7975) -> (202.7525, -102.8025)
  line L362 (202.7525, -102.8025) -> (188.7475, -102.8025)
  line L363 (188.7475, -102.8025) -> (188.7475, -88.7975)
  line L364 (188.7475, -88.7975) -> (202.7525, -102.8025) construction
  line L365 (202.7525, -88.7975) -> (188.7475, -102.8025) construction
  line L366 (15.9975, -107.8975) -> (30.0025, -107.8975)
  line L367 (30.0025, -107.8975) -> (30.0025, -121.9025)
  line L368 (30.0025, -121.9025) -> (15.9975, -121.9025)
  line L369 (15.9975, -121.9025) -> (15.9975, -107.8975)
  line L370 (15.9975, -107.8975) -> (30.0025, -121.9025) construction
  line L371 (30.0025, -107.8975) -> (15.9975, -121.9025) construction
  line L372 (40.4975, -107.8975) -> (54.5025, -107.8975)
  line L373 (54.5025, -107.8975) -> (54.5025, -121.9025)
  line L374 (54.5025, -121.9025) -> (40.4975, -121.9025)
  line L375 (40.4975, -121.9025) -> (40.4975, -107.8975)
  line L376 (40.4975, -107.8975) -> (54.5025, -121.9025) construction
  line L377 (54.5025, -107.8975) -> (40.4975, -121.9025) construction
  line L378 (210, -1.9975) -> (0, -1.9975)
  line L379 (0, -1.9975) -> (0, -122.9025)
  line L380 (0, -122.9025) -> (216.3009, -122.9025)
  line L381 (5, -50.5975) -> (11, -50.5975)
  line L382 (11, -50.5975) -> (11, -62.7975)
  line L383 (11, -62.7975) -> (5, -62.7975)
  line L384 (5, -62.7975) -> (5, -50.5975)
  line L385 (29, -50.5975) -> (35, -50.5975)
  line L386 (35, -50.5975) -> (35, -62.7975)
  line L387 (35, -62.7975) -> (29, -62.7975)
  line L388 (29, -62.7975) -> (29, -50.5975)
  line L389 (8, -50.5975) -> (8, -62.7975) construction
  line L390 (32, -50.5975) -> (32, -62.7975) construction
  line L391 (200.6018, -107.9725) -> (206.6018, -107.9725)
  line L392 (206.6018, -107.9725) -> (206.6018, -120.1725)
  line L393 (206.6018, -120.1725) -> (200.6018, -120.1725)
  line L394 (200.6018, -120.1725) -> (200.6018, -107.9725)
  line L395 (67.1018, -107.9725) -> (73.1017, -107.9725)
  line L396 (73.1017, -107.9725) -> (73.1018, -120.1725)
  line L397 (73.1018, -120.1725) -> (67.1018, -120.1725)
  line L398 (67.1018, -120.1725) -> (67.1018, -107.9725)
  line L399 (70.1018, -107.9725) -> (70.1018, -120.1725) construction
  line L400 (203.6018, -107.9725) -> (203.6018, -120.1725) construction
  line L401 (119.75, -21.25) -> (163.5, -21.25)
  line L402 (163.5, -21.25) -> (163.5, -28.75)
  line L403 (163.5, -28.75) -> (119.75, -28.75)
  line L404 (119.75, -28.75) -> (119.75, -21.25)
  point P0 (0, 0)
  dimension "d0" = 14.005
  dimension "d1" = 14.005
  dimension "d3" = 14.005
  dimension "d4" = 14.005
  dimension "d5" = 14.005
  dimension "d6" = 14.005
  dimension "d7" = 14.005
  dimension "d8" = 14.005
  dimension "d9" = 14.005
  dimension "d10" = 14.005
  dimension "d11" = 14.005
  dimension "d12" = 14.005
  dimension "d13" = 14.005
  dimension "d14" = 14.005
  dimension "d15" = 14.005
  dimension "d16" = 14.005
  dimension "d17" = 14.005
  dimension "d18" = 14.005
  dimension "d19" = 14.005
  dimension "d20" = 14.005
  dimension "d21" = 14.005
  dimension "d22" = 14.005
  dimension "d23" = 14.005
  dimension "d24" = 14.005
  dimension "d25" = 14.005
  dimension "d26" = 14.005
  dimension "d27" = 14.005
  dimension "d28" = 14.005
  dimension "d29" = 14.005
  dimension "d30" = 14.005
  dimension "d31" = 14.005
  dimension "d32" = 14.005
  dimension "d33" = 14.005
  dimension "d34" = 14.005
  dimension "d35" = 14.005
  dimension "d36" = 14.005
  dimension "d37" = 14.005
  dimension "d38" = 14.005
  dimension "d39" = 14.005
  dimension "d40" = 14.005
  dimension "d41" = 14.005
  dimension "d42" = 14.005
  dimension "d43" = 14.005
  dimension "d44" = 14.005
  dimension "d45" = 14.005
  dimension "d46" = 14.005
  dimension "d47" = 14.005
  dimension "d48" = 14.005
  dimension "d49" = 14.005
  dimension "d50" = 14.005
  dimension "d51" = 14.005
  dimension "d52" = 14.005
  dimension "d53" = 14.005
  dimension "d54" = 14.005
  dimension "d55" = 14.005
  dimension "d56" = 14.005
  dimension "d57" = 14.005
  dimension "d58" = 14.005
  dimension "d59" = 14.005
  dimension "d60" = 14.005
  dimension "d61" = 14.005
  dimension "d62" = 14.005
  dimension "d63" = 14.005
  dimension "d64" = 14.005
  constraints: 754 end point, 117 midpoint, 117 parallel, 83 perpendicular, 60 horizontal, 25 point on line, 19 collinear, 1 vertical
  measures "d0" distance of L60.end L61.end
  measures "d1" distance of L59.end L60.end
  measures "d3" distance of L66.end L67.end
  measures "d4" distance of L65.end L66.end
  measures "d5" distance of L73.end L74.end
  measures "d6" distance of L72.end L73.end
  measures "d7" distance of L79.end L80.end
  measures "d8" distance of L78.end L79.end
  measures "d9" distance of L85.end L86.end
  measures "d10" distance of L84.end L85.end
  measures "d11" distance of L91.end L92.end
  measures "d12" distance of L90.end L91.end
  measures "d13" distance of L97.end L98.end
  measures "d14" distance of L96.end L97.end
  measures "d15" distance of L103.end L104.end
  measures "d16" distance of L102.end L103.end
  measures "d17" distance of L109.end L110.end
  measures "d18" distance of L108.end L109.end
  measures "d19" distance of L115.end L116.end
  measures "d20" distance of L114.end L115.end
  measures "d21" distance of L121.end L122.end
  measures "d22" distance of L120.end L121.end
  measures "d23" distance of L127.end L128.end
  measures "d24" distance of L126.end L127.end
  measures "d25" distance of L133.end L134.end
  measures "d26" distance of L132.end L133.end
  measures "d27" distance of L139.end L140.end
  measures "d28" distance of L138.end L139.end
  measures "d29" distance of L145.end L146.end
  measures "d30" distance of L144.end L145.end
  measures "d31" distance of L151.end L152.end
  measures "d32" distance of L150.end L151.end
  measures "d33" distance of L157.end L158.end
  measures "d34" distance of L156.end L157.end
  measures "d35" distance of L163.end L164.end
  measures "d36" distance of L162.end L163.end
  measures "d37" distance of L169.end L170.end
  measures "d38" distance of L168.end L169.end
  measures "d39" distance of L175.end L176.end
  measures "d40" distance of L174.end L175.end
  measures "d41" distance of L181.end L182.end
  measures "d42" distance of L180.end L181.end
  measures "d43" distance of L187.end L188.end
  measures "d44" distance of L186.end L187.end
  measures "d45" distance of L193.end L194.end
  measures "d46" distance of L192.end L193.end
  measures "d47" distance of L199.end L200.end
  measures "d48" distance of L198.end L199.end
  measures "d49" distance of L205.end L206.end
  measures "d50" distance of L204.end L205.end
  measures "d51" distance of L211.end L212.end
  measures "d52" distance of L210.end L211.end
  measures "d53" distance of L217.end L218.end
  measures "d54" distance of L216.end L217.end
  measures "d55" distance of L223.end L224.end
  measures "d56" distance of L222.end L223.end
  measures "d57" distance of L229.end L230.end
  measures "d58" distance of L228.end L229.end
  measures "d59" distance of L235.end L236.end
  measures "d60" distance of L234.end L235.end
  measures "d61" distance of L241.end L242.end
  measures "d62" distance of L240.end L241.end
  measures "d63" distance of L247.end L248.end
  measures "d64" distance of L246.end L247.end
extrude "Extrusion1" add sketch "Sketch3" along normal blind 0.5